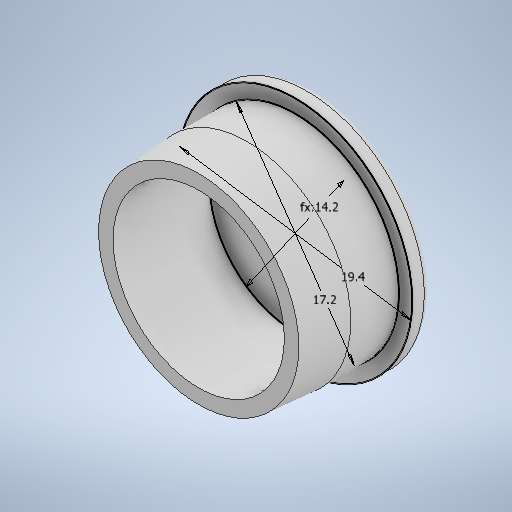
# Autodesk Inventor part: Rodend19mil
Saved by Autodesk Inventor 2025.2 (Build 292293000, 293)
## iProperties
Created: 2025-02-25
Part Number: Rodend19mil
Material: Generic
Document SubType Name: Modeling
Designer: cutterj
Density: 1 g/cm^3
Appearance: Default
Author: cutterj
Autodesk Inventor part; units mm, degrees
ref_plane "YZ Plane" through (0, 0, 0) normal (1, 0, 0) x (0, 1, 0)
ref_plane "XZ Plane" through (0, 0, 0) normal (0, 1, 0) x (-1, 0, 0)
ref_plane "XY Plane" through (0, 0, 0) normal (0, 0, 1) x (1, 0, 0)
sketch "Sketch1" plane through (0, 0, 0) normal (0, 0, 1) x (1, 0, 0)
  circle A0 centre (0, 0) radius 9.7
  circle A1 centre (0, 0) radius 8.6
  circle A2 centre (0, 0) radius 7.1
  dimension "d0" = 19.4
  dimension "d1" = 17.2
  dimension "d6" = 14.2
  constraints: 3 centre point, 3 coincident
  measures "d0" diameter of A0
  measures "d1" diameter of A1
  measures "d6" diameter of A2
extrude "Extrusion1" add sketch "Sketch1" along normal blind 8 contours A1 | A2
extrude "Extrusion2" add sketch "Sketch1" against normal blind 1.5 contours A0 | A1 | A2
extrude "Extrusion3" cut sketch "Sketch1" along normal up to next contours A2
fillet "Fillet1" radius 0.5 1 edges at (-9.7, 0, -1.5)
chamfer "Chamfer1" distance 0.3 distance2 4 1 edges at (-8.6, 0, 8) measured on face at (7.9479, -1.2524, 8)
body "Solid1"
